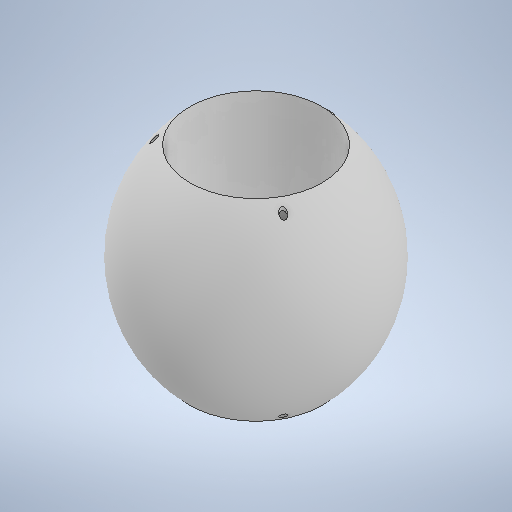
# Autodesk Inventor part: Buoy 12 7inx1in shpere
Saved by Autodesk Inventor 2025 (Build 290162000, 162)
## iProperties
Created: 2024-07-18
Part Number: Buoy 12 7inx1in shpere
Material: Generic
Document SubType Name: Modeling
Designer: track
Mass: 2545.06 g
Surface Area: 1978.43 cm^2
Volume: 2545.06 cm^3
Density: 1 g/cm^3
Appearance: Default
Author: track
## iProperties of the stored document Buoy 11 8inx1in shpere_3DPrint.ipt
Created: 2024-07-18
Part Number: Buoy 11 8inx1in shpere_3DPrint
Material: Generic
Document SubType Name: Modeling
Designer: track
Density: 1 g/cm^3
Appearance: Default
Author: track
Autodesk Inventor part; units mm, degrees
ref_plane "YZ Plane" through (0, 0, 0) normal (1, 0, 0) x (0, 1, 0)
ref_plane "XZ Plane" through (0, 0, 0) normal (0, 1, 0) x (-1, 0, 0)
ref_plane "XY Plane" through (0, 0, 0) normal (0, 0, 1) x (1, 0, 0)
sketch "Sketch1" plane through (0, 0, 0) normal (0, 0, 1) x (1, 0, 0)
  line L0 (0, 0) -> (0, 177.8) construction
  line L1 (0, 177.8) -> (60.96, 177.8) construction
  line L2 (60.96, 177.8) -> (60.96, 0)
  line L3 (60.96, 0) -> (0, 0) construction
  arc A0 (60.96, 0) -> (60.96, 177.8) centre (-23.7067, 88.9) ccw
  line L4 (99.06, 88.9) -> (60.96, 88.9) construction
  line L5 (62.96, 4.796) -> (62.96, 173.004)
  arc A1 (62.96, 4.796) -> (62.96, 173.004) centre (-23.7067, 88.9) ccw
  dimension "d0" = 60.96
  dimension "d1" = 177.8
  dimension "d2" = 38.1
  dimension "d3" = 2
  constraints: 12 end point, 5 point on circle, 3 perpendicular, 2 centre point, 1 midpoint, 1 vertical, 1 other
  measures "d0" distance of L0.end L1.end
  measures "d1" distance of L0.start L0.end
  measures "d2" distance of L4.start L4.end
  measures "d3" distance between parallel lines of L2 L5
revolve "Revolution1" add sketch "Sketch1" angle 360 about axis through (0, 0, 0) along (0, 1, 0)
sketch "Sketch2" plane through (0, 0, 0) normal (0, 1, 0) x (-1, 0, 0)
  line L0 (0, 0) -> (0, -68.58)
  circle A0 centre (0, -68.58) radius 3
  dimension "d5" = 6
  dimension "d6" = 68.58
  constraints: 2 end point, 1 centre point, 1 coincident, 1 vertical
  measures "d5" diameter of A0
  measures "d6" distance of L0.start L0.end
extrude "Extrusion1" cut sketch "Sketch2" along normal through all
pattern_circular "Circular Pattern1" count 3 over 360 about axis through (0, 88.9, 0) along (0, 1, 0) of "Extrusion1"
body "Solid1"
